Autodesk Fusion 360 part; units mm, degrees
(part 4 of 14)
  arc A924 (85.1535, 49.2252) -> (85.2805, 49.2252) centre (85.217, 49.2252) ccw
  line L1593 (84.034, 50.673) -> (84.584, 50.673)
  arc A925 (84.2645, 50.9778) -> (84.1375, 50.9778) centre (84.201, 50.9778) ccw
  arc A926 (84.2645, 50.9778) -> (84.1375, 50.9778) centre (84.201, 50.9778) ccw
  line L1594 (84.834, 50.9778) -> (84.584, 50.9778)
  line L1595 (84.834, 50.673) -> (85.384, 50.673)
  line L1596 (85.217, 50.9778) -> (85.217, 50.3682)
  arc A927 (84.2645, 49.2252) -> (84.1375, 49.2252) centre (84.201, 49.2252) ccw
  arc A928 (84.1588, 49.23) -> (84.1592, 49.23) centre (84.159, 49.23) ccw
  arc A929 (84.1375, 50.9778) -> (84.2645, 50.9778) centre (84.201, 50.9778) ccw
  arc A930 (85.2805, 50.3682) -> (85.1535, 50.3682) centre (85.217, 50.3682) ccw
  line L1597 (85.259, 49.83) -> (84.159, 49.83)
  arc A931 (85.2805, 49.2252) -> (85.1535, 49.2252) centre (85.217, 49.2252) ccw
  line L1598 (84.034, 50.673) -> (84.584, 50.673)
  line L1599 (84.834, 49.8348) -> (84.584, 49.8348)
  line L1600 (85.259, 49.23) -> (85.259, 49.83)
  line L1601 (84.159, 49.83) -> (84.159, 49.23)
  line L1602 (84.584, 49.2252) -> (84.834, 49.2252)
  line L1603 (84.834, 50.673) -> (85.384, 50.673)
  arc A932 (85.2588, 49.83) -> (85.2592, 49.83) centre (85.259, 49.83) ccw
  line L1604 (84.201, 49.2252) -> (84.201, 49.8348)
  line L1605 (84.034, 49.53) -> (84.584, 49.53)
  arc A933 (84.2645, 50.3682) -> (84.1375, 50.3682) centre (84.201, 50.3682) ccw
  line L1606 (84.584, 50.9778) -> (84.584, 50.3682)
  line L1607 (84.201, 50.9778) -> (85.217, 50.9778)
  arc A934 (84.2645, 50.3682) -> (84.1375, 50.3682) centre (84.201, 50.3682) ccw
  arc A935 (84.1375, 50.3682) -> (84.2645, 50.3682) centre (84.201, 50.3682) ccw
  line L1608 (84.834, 50.3682) -> (84.834, 50.9778)
  arc A936 (84.1375, 49.8348) -> (84.2645, 49.8348) centre (84.201, 49.8348) ccw
  line L1609 (84.034, 49.53) -> (84.584, 49.53)
  arc A937 (85.2805, 50.3682) -> (85.1535, 50.3682) centre (85.217, 50.3682) ccw
  line L1610 (85.217, 49.2252) -> (84.201, 49.2252)
  line L1611 (85.217, 50.3682) -> (84.201, 50.3682)
  line L1612 (84.201, 49.8348) -> (85.217, 49.8348)
  arc A938 (84.1375, 49.2252) -> (84.2645, 49.2252) centre (84.201, 49.2252) ccw
  line L1613 (85.217, 49.8348) -> (85.217, 49.2252)
  arc A939 (84.1588, 49.83) -> (84.1592, 49.83) centre (84.159, 49.83) ccw
  line L1614 (84.834, 50.673) -> (85.384, 50.673)
  line L1615 (84.201, 50.3682) -> (84.201, 50.9778)
  arc A940 (84.1375, 50.9778) -> (84.2645, 50.9778) centre (84.201, 50.9778) ccw
  line L1616 (84.584, 50.3682) -> (84.834, 50.3682)
  arc A941 (85.2805, 49.2252) -> (85.1535, 49.2252) centre (85.217, 49.2252) ccw
  arc A942 (85.1535, 50.3682) -> (85.2805, 50.3682) centre (85.217, 50.3682) ccw
  line L1617 (84.201, 49.8348) -> (85.217, 49.8348)
  arc A943 (84.1592, 49.83) -> (84.1588, 49.83) centre (84.159, 49.83) ccw
  arc A944 (85.2805, 49.8348) -> (85.1535, 49.8348) centre (85.217, 49.8348) ccw
  line L1618 (85.217, 49.8348) -> (85.217, 49.2252)
  line L1619 (84.834, 49.53) -> (85.384, 49.53)
  arc A945 (85.1535, 50.9778) -> (85.2805, 50.9778) centre (85.217, 50.9778) ccw
  arc A946 (85.1535, 49.8348) -> (85.2805, 49.8348) centre (85.217, 49.8348) ccw
  arc A947 (80.818, 55.5408) -> (80.818, 55.5412) centre (80.818, 55.541) ccw
  line L1620 (84.834, 49.53) -> (85.384, 49.53)
  line L1621 (80.518, 54.316) -> (80.518, 54.866)
  line L1622 (80.218, 54.441) -> (80.818, 54.441)
  arc A948 (85.2592, 49.83) -> (85.2588, 49.83) centre (85.259, 49.83) ccw
  arc A949 (80.2132, 54.5465) -> (80.2132, 54.4195) centre (80.2132, 54.483) ccw
  arc A950 (80.8228, 55.4355) -> (80.8228, 55.5625) centre (80.8228, 55.499) ccw
  line L1623 (80.8228, 55.499) -> (80.8228, 54.483)
  line L1624 (80.518, 55.116) -> (80.518, 55.666)
  line L1625 (79.6798, 55.499) -> (79.6798, 54.483)
  arc A951 (80.8228, 55.5625) -> (80.8228, 55.4355) centre (80.8228, 55.499) ccw
  arc A952 (80.218, 55.5408) -> (80.218, 55.5412) centre (80.218, 55.541) ccw
  arc A953 (80.8228, 54.4195) -> (80.8228, 54.5465) centre (80.8228, 54.483) ccw
  arc A954 (80.218, 54.4408) -> (80.218, 54.4412) centre (80.218, 54.441) ccw
  line L1626 (80.8228, 54.866) -> (80.8228, 55.116)
  line L1627 (80.8228, 54.483) -> (80.2132, 54.483)
  arc A955 (80.2132, 54.4195) -> (80.2132, 54.5465) centre (80.2132, 54.483) ccw
  line L1628 (84.834, 49.53) -> (85.384, 49.53)
  arc A956 (80.818, 55.5412) -> (80.818, 55.5408) centre (80.818, 55.541) ccw
  line L1629 (80.218, 55.541) -> (80.218, 54.441)
  line L1630 (79.0702, 55.499) -> (79.6798, 55.499)
  arc A957 (79.6798, 54.5465) -> (79.6798, 54.4195) centre (79.6798, 54.483) ccw
  arc A958 (80.2132, 55.5625) -> (80.2132, 55.4355) centre (80.2132, 55.499) ccw
  line L1631 (79.675, 54.441) -> (79.675, 55.541)
  arc A959 (79.675, 54.4408) -> (79.675, 54.4412) centre (79.675, 54.441) ccw
  line L1632 (79.6798, 54.483) -> (79.0702, 54.483)
  arc A960 (85.1535, 49.2252) -> (85.2805, 49.2252) centre (85.217, 49.2252) ccw
  arc A961 (80.2132, 55.4355) -> (80.2132, 55.5625) centre (80.2132, 55.499) ccw
  line L1633 (80.2132, 54.483) -> (80.2132, 55.499)
  arc A962 (80.8228, 54.4195) -> (80.8228, 54.5465) centre (80.8228, 54.483) ccw
  arc A963 (80.8228, 55.5625) -> (80.8228, 55.4355) centre (80.8228, 55.499) ccw
  arc A964 (80.2132, 54.4195) -> (80.2132, 54.5465) centre (80.2132, 54.483) ccw
  line L1634 (84.834, 49.2252) -> (84.834, 49.8348)
  line L1635 (80.8228, 55.499) -> (80.8228, 54.483)
  line L1636 (80.8228, 55.116) -> (80.2132, 55.116)
  arc A965 (85.1535, 49.8348) -> (85.2805, 49.8348) centre (85.217, 49.8348) ccw
  arc A966 (80.218, 55.5412) -> (80.218, 55.5408) centre (80.218, 55.541) ccw
  arc A967 (80.8228, 54.5465) -> (80.8228, 54.4195) centre (80.8228, 54.483) ccw
  arc A968 (80.2132, 54.5465) -> (80.2132, 54.4195) centre (80.2132, 54.483) ccw
  line L1637 (80.2132, 55.499) -> (80.8228, 55.499)
  arc A969 (84.2645, 49.2252) -> (84.1375, 49.2252) centre (84.201, 49.2252) ccw
  arc A970 (84.2645, 49.8348) -> (84.1375, 49.8348) centre (84.201, 49.8348) ccw
  line L1638 (80.818, 55.541) -> (80.218, 55.541)
  arc A971 (80.818, 54.4408) -> (80.818, 54.4412) centre (80.818, 54.441) ccw
  arc A972 (80.2132, 55.5625) -> (80.2132, 55.4355) centre (80.2132, 55.499) ccw
  line L1639 (80.518, 54.316) -> (80.518, 54.866)
  line L1640 (80.2132, 55.499) -> (80.8228, 55.499)
  line L1641 (80.518, 54.316) -> (80.518, 54.866)
  arc A973 (80.218, 54.4412) -> (80.218, 54.4408) centre (80.218, 54.441) ccw
  line L1642 (80.2132, 54.483) -> (80.2132, 55.499)
  arc A974 (84.2645, 49.8348) -> (84.1375, 49.8348) centre (84.201, 49.8348) ccw
  arc A975 (80.818, 54.4412) -> (80.818, 54.4408) centre (80.818, 54.441) ccw
  line L1643 (80.2132, 54.866) -> (80.8228, 54.866)
  arc A976 (79.0702, 55.4355) -> (79.0702, 55.5625) centre (79.0702, 55.499) ccw
  line L1644 (80.2132, 55.116) -> (80.2132, 54.866)
  arc A977 (80.2132, 55.4355) -> (80.2132, 55.5625) centre (80.2132, 55.499) ccw
  line L1645 (84.159, 49.23) -> (85.259, 49.23)
  arc A978 (84.1592, 49.23) -> (84.1588, 49.23) centre (84.159, 49.23) ccw
  line L1646 (80.8228, 54.483) -> (80.2132, 54.483)
  line L1647 (85.217, 49.2252) -> (84.201, 49.2252)
  arc A979 (85.2805, 49.8348) -> (85.1535, 49.8348) centre (85.217, 49.8348) ccw
  arc A980 (80.8228, 55.4355) -> (80.8228, 55.5625) centre (80.8228, 55.499) ccw
  line L1648 (80.818, 54.441) -> (80.818, 55.541)
  arc A981 (80.8228, 54.5465) -> (80.8228, 54.4195) centre (80.8228, 54.483) ccw
  line L1649 (79.375, 55.116) -> (79.375, 55.666)
  arc A982 (76.1365, 50.3682) -> (76.2635, 50.3682) centre (76.2, 50.3682) ccw
  line L1650 (80.518, 55.116) -> (80.518, 55.666)
  line L1651 (77.258, 50.973) -> (76.158, 50.973)
  arc A983 (79.6798, 55.5625) -> (79.6798, 55.4355) centre (79.6798, 55.499) ccw
  arc A984 (79.075, 54.4412) -> (79.075, 54.4408) centre (79.075, 54.441) ccw
  line L1652 (76.583, 50.3682) -> (76.833, 50.3682)
  arc A985 (77.1525, 50.9778) -> (77.2795, 50.9778) centre (77.216, 50.9778) ccw
  arc A986 (76.1365, 50.9778) -> (76.2635, 50.9778) centre (76.2, 50.9778) ccw
  arc A987 (76.2635, 50.3682) -> (76.1365, 50.3682) centre (76.2, 50.3682) ccw
  arc A988 (79.075, 55.5408) -> (79.075, 55.5412) centre (79.075, 55.541) ccw
  arc A989 (76.2635, 50.3682) -> (76.1365, 50.3682) centre (76.2, 50.3682) ccw
  arc A990 (79.675, 54.4412) -> (79.675, 54.4408) centre (79.675, 54.441) ccw
  line L1653 (76.833, 50.3682) -> (76.833, 50.9778)
  arc A991 (79.0702, 54.4195) -> (79.0702, 54.5465) centre (79.0702, 54.483) ccw
  arc A992 (79.0702, 54.5465) -> (79.0702, 54.4195) centre (79.0702, 54.483) ccw
  line L1654 (76.833, 50.9778) -> (76.583, 50.9778)
  arc A993 (77.2795, 50.3682) -> (77.1525, 50.3682) centre (77.216, 50.3682) ccw
  line L1655 (77.216, 50.3682) -> (76.2, 50.3682)
  arc A994 (77.2578, 50.973) -> (77.2582, 50.973) centre (77.258, 50.973) ccw
  arc A995 (77.2582, 50.373) -> (77.2578, 50.373) centre (77.258, 50.373) ccw
  arc A996 (76.2635, 50.9778) -> (76.1365, 50.9778) centre (76.2, 50.9778) ccw
  arc A997 (76.1582, 50.373) -> (76.1578, 50.373) centre (76.158, 50.373) ccw
  line L1656 (76.583, 50.9778) -> (76.583, 50.3682)
  line L1657 (76.2, 50.9778) -> (77.216, 50.9778)
  arc A998 (76.1365, 50.3682) -> (76.2635, 50.3682) centre (76.2, 50.3682) ccw
  line L1658 (79.6798, 54.483) -> (79.0702, 54.483)
  arc A999 (79.6798, 55.4355) -> (79.6798, 55.5625) centre (79.6798, 55.499) ccw
  line L1659 (79.0702, 54.483) -> (79.0702, 55.499)
  arc A1000 (79.6798, 54.4195) -> (79.6798, 54.5465) centre (79.6798, 54.483) ccw
  line L1660 (76.2, 50.9778) -> (77.216, 50.9778)
  arc A1001 (79.0702, 55.5625) -> (79.0702, 55.4355) centre (79.0702, 55.499) ccw
  line L1661 (79.0702, 54.866) -> (79.6798, 54.866)
  arc A1002 (77.2582, 50.973) -> (77.2578, 50.973) centre (77.258, 50.973) ccw
  line L1662 (79.0702, 55.116) -> (79.0702, 54.866)
  arc A1003 (79.0702, 54.5465) -> (79.0702, 54.4195) centre (79.0702, 54.483) ccw
  arc A1004 (79.675, 55.5412) -> (79.675, 55.5408) centre (79.675, 55.541) ccw
  arc A1005 (79.0702, 55.5625) -> (79.0702, 55.4355) centre (79.0702, 55.499) ccw
  line L1663 (77.216, 50.9778) -> (77.216, 50.3682)
  arc A1006 (77.1525, 50.3682) -> (77.2795, 50.3682) centre (77.216, 50.3682) ccw
  line L1664 (79.675, 55.541) -> (79.075, 55.541)
  arc A1007 (79.0702, 54.4195) -> (79.0702, 54.5465) centre (79.0702, 54.483) ccw
  arc A1008 (79.6798, 54.4195) -> (79.6798, 54.5465) centre (79.6798, 54.483) ccw
  arc A1009 (79.075, 55.5412) -> (79.075, 55.5408) centre (79.075, 55.541) ccw
  line L1665 (79.375, 54.316) -> (79.375, 54.866)
  line L1666 (79.075, 54.441) -> (79.675, 54.441)
  arc A1010 (77.2578, 50.373) -> (77.2582, 50.373) centre (77.258, 50.373) ccw
  line L1667 (76.158, 50.373) -> (77.258, 50.373)
  line L1668 (79.375, 55.116) -> (79.375, 55.666)
  arc A1011 (77.2795, 50.9778) -> (77.1525, 50.9778) centre (77.216, 50.9778) ccw
  line L1669 (79.6798, 55.499) -> (79.6798, 54.483)
  line L1670 (79.6798, 54.866) -> (79.6798, 55.116)
  arc A1012 (79.6798, 55.5625) -> (79.6798, 55.4355) centre (79.6798, 55.499) ccw
  arc A1013 (79.0702, 55.4355) -> (79.0702, 55.5625) centre (79.0702, 55.499) ccw
  arc A1014 (79.075, 54.4408) -> (79.075, 54.4412) centre (79.075, 54.441) ccw
  line L1671 (79.6798, 55.116) -> (79.0702, 55.116)
  arc A1015 (79.6798, 54.5465) -> (79.6798, 54.4195) centre (79.6798, 54.483) ccw
  line L1672 (79.075, 55.541) -> (79.075, 54.441)
  line L1673 (79.0702, 54.483) -> (79.0702, 55.499)
  line L1674 (79.0702, 55.499) -> (79.6798, 55.499)
  line L1675 (80.518, 55.116) -> (80.518, 55.666)
  arc A1016 (79.675, 55.5408) -> (79.675, 55.5412) centre (79.675, 55.541) ccw
  arc A1017 (76.2635, 50.9778) -> (76.1365, 50.9778) centre (76.2, 50.9778) ccw
  arc A1018 (79.6798, 55.4355) -> (79.6798, 55.5625) centre (79.6798, 55.499) ccw
  line L1676 (26.999, 28.694) -> (26.399, 28.694)
  arc A1019 (76.1578, 50.373) -> (76.1582, 50.373) centre (76.158, 50.373) ccw
  arc A1020 (26.399, 28.6943) -> (26.399, 28.6938) centre (26.399, 28.694) ccw
  line L1677 (77.216, 50.3682) -> (76.2, 50.3682)
  line L1678 (79.375, 54.316) -> (79.375, 54.866)
  line L1679 (77.216, 50.9778) -> (77.216, 50.3682)
  line L1680 (26.3942, 27.636) -> (26.3942, 28.652)
  arc A1021 (26.999, 27.5938) -> (26.999, 27.5943) centre (26.999, 27.594) ccw
  arc A1022 (26.399, 27.5938) -> (26.399, 27.5943) centre (26.399, 27.594) ccw
  line L1681 (27.0038, 27.636) -> (26.3942, 27.636)
  arc A1023 (26.999, 28.6938) -> (26.999, 28.6943) centre (26.999, 28.694) ccw
  line L1682 (26.3942, 28.652) -> (27.0038, 28.652)
  line L1683 (76.583, 50.673) -> (76.033, 50.673)
  arc A1024 (27.0038, 27.5725) -> (27.0038, 27.6995) centre (27.0038, 27.636) ccw
  arc A1025 (27.0038, 27.6995) -> (27.0038, 27.5725) centre (27.0038, 27.636) ccw
  line L1684 (26.3942, 28.269) -> (26.3942, 28.019)
  arc A1026 (26.399, 28.6938) -> (26.399, 28.6943) centre (26.399, 28.694) ccw
  line L1685 (82.804, 30.4038) -> (83.82, 30.4038)
  line L1686 (76.583, 50.673) -> (76.033, 50.673)
  arc A1027 (26.3942, 28.5885) -> (26.3942, 28.7155) centre (26.3942, 28.652) ccw
  line L1687 (79.375, 55.116) -> (79.375, 55.666)
  line L1688 (26.999, 27.594) -> (26.999, 28.694)
  line L1689 (26.3942, 28.652) -> (27.0038, 28.652)
  line L1690 (26.399, 27.594) -> (26.999, 27.594)
  line L1691 (26.3942, 27.636) -> (26.3942, 28.652)
  line L1692 (26.699, 28.269) -> (26.699, 28.819)
  arc A1028 (26.3942, 27.5725) -> (26.3942, 27.6995) centre (26.3942, 27.636) ccw
  arc A1029 (83.8622, 29.799) -> (83.8618, 29.799) centre (83.862, 29.799) ccw
  arc A1030 (26.3942, 27.5725) -> (26.3942, 27.6995) centre (26.3942, 27.636) ccw
  line L1693 (76.158, 50.973) -> (76.158, 50.373)
  line L1694 (27.0038, 27.636) -> (26.3942, 27.636)
  arc A1031 (76.1578, 50.973) -> (76.1582, 50.973) centre (76.158, 50.973) ccw
  arc A1032 (27.0038, 28.5885) -> (27.0038, 28.7155) centre (27.0038, 28.652) ccw
  line L1695 (77.383, 50.673) -> (76.833, 50.673)
  line L1696 (76.2, 50.3682) -> (76.2, 50.9778)
  arc A1033 (26.3942, 27.6995) -> (26.3942, 27.5725) centre (26.3942, 27.636) ccw
  arc A1034 (83.8618, 29.799) -> (83.8622, 29.799) centre (83.862, 29.799) ccw
  arc A1035 (77.1525, 50.3682) -> (77.2795, 50.3682) centre (77.216, 50.3682) ccw
  arc A1036 (76.1365, 50.9778) -> (76.2635, 50.9778) centre (76.2, 50.9778) ccw
  arc A1037 (77.2795, 50.3682) -> (77.1525, 50.3682) centre (77.216, 50.3682) ccw
  arc A1038 (26.999, 28.6943) -> (26.999, 28.6938) centre (26.999, 28.694) ccw
  arc A1039 (26.3942, 28.5885) -> (26.3942, 28.7155) centre (26.3942, 28.652) ccw
  arc A1040 (26.999, 27.5943) -> (26.999, 27.5938) centre (26.999, 27.594) ccw
  arc A1041 (26.3942, 28.7155) -> (26.3942, 28.5885) centre (26.3942, 28.652) ccw
  line L1697 (76.583, 50.673) -> (76.033, 50.673)
  line L1698 (26.3942, 28.019) -> (27.0038, 28.019)
  line L1699 (79.375, 54.316) -> (79.375, 54.866)
  arc A1042 (77.1525, 50.9778) -> (77.2795, 50.9778) centre (77.216, 50.9778) ccw
  arc A1043 (27.0038, 27.6995) -> (27.0038, 27.5725) centre (27.0038, 27.636) ccw
  line L1700 (77.383, 50.673) -> (76.833, 50.673)
  arc A1044 (27.0038, 28.5885) -> (27.0038, 28.7155) centre (27.0038, 28.652) ccw
  arc A1045 (76.1582, 50.973) -> (76.1578, 50.973) centre (76.158, 50.973) ccw
  arc A1046 (77.2795, 50.9778) -> (77.1525, 50.9778) centre (77.216, 50.9778) ccw
  arc A1047 (26.399, 27.5943) -> (26.399, 27.5938) centre (26.399, 27.594) ccw
  arc A1048 (27.0038, 27.5725) -> (27.0038, 27.6995) centre (27.0038, 27.636) ccw
  line L1701 (27.0038, 28.652) -> (27.0038, 27.636)
  line L1702 (76.2, 50.3682) -> (76.2, 50.9778)
  line L1703 (26.399, 28.694) -> (26.399, 27.594)
  line L1704 (27.0038, 28.652) -> (27.0038, 27.636)
  line L1705 (77.383, 50.673) -> (76.833, 50.673)
  arc A1049 (26.3942, 28.7155) -> (26.3942, 28.5885) centre (26.3942, 28.652) ccw
  line L1706 (77.258, 50.373) -> (77.258, 50.973)
  arc A1050 (27.0038, 28.7155) -> (27.0038, 28.5885) centre (27.0038, 28.652) ccw
  arc A1051 (27.0038, 28.7155) -> (27.0038, 28.5885) centre (27.0038, 28.652) ccw
  line L1707 (28.1468, 28.652) -> (28.1468, 27.636)
  line L1708 (28.142, 27.594) -> (28.142, 28.694)
  line L1709 (27.542, 28.694) -> (27.542, 27.594)
  line L1710 (82.637, 30.099) -> (83.187, 30.099)
  arc A1052 (82.8675, 29.7942) -> (82.7405, 29.7942) centre (82.804, 29.7942) ccw
  line L1711 (83.187, 30.4038) -> (83.187, 29.7942)
  arc A1053 (82.8675, 30.4038) -> (82.7405, 30.4038) centre (82.804, 30.4038) ccw
  line L1712 (83.82, 29.7942) -> (82.804, 29.7942)
  line L1713 (27.542, 27.594) -> (28.142, 27.594)
  line L1714 (83.82, 29.7942) -> (82.804, 29.7942)
  arc A1054 (83.8618, 30.399) -> (83.8622, 30.399) centre (83.862, 30.399) ccw
  arc A1055 (82.7622, 29.799) -> (82.7618, 29.799) centre (82.762, 29.799) ccw
  line L1715 (83.437, 30.099) -> (83.987, 30.099)
  line L1716 (83.437, 30.099) -> (83.987, 30.099)
  line L1717 (83.437, 30.4038) -> (83.187, 30.4038)
  arc A1056 (83.7565, 29.7942) -> (83.8835, 29.7942) centre (83.82, 29.7942) ccw
  arc A1057 (26.3942, 27.6995) -> (26.3942, 27.5725) centre (26.3942, 27.636) ccw
  arc A1058 (83.7565, 29.7942) -> (83.8835, 29.7942) centre (83.82, 29.7942) ccw
  arc A1059 (82.8675, 29.7942) -> (82.7405, 29.7942) centre (82.804, 29.7942) ccw
  line L1718 (83.82, 30.4038) -> (83.82, 29.7942)
  line L1719 (26.699, 27.469) -> (26.699, 28.019)
  arc A1060 (83.7565, 30.4038) -> (83.8835, 30.4038) centre (83.82, 30.4038) ccw
  line L1720 (26.699, 28.269) -> (26.699, 28.819)
  line L1721 (27.0038, 28.269) -> (26.3942, 28.269)
  line L1722 (83.82, 30.4038) -> (83.82, 29.7942)
  arc A1061 (82.7405, 29.7942) -> (82.8675, 29.7942) centre (82.804, 29.7942) ccw
  arc A1062 (83.7565, 30.4038) -> (83.8835, 30.4038) centre (83.82, 30.4038) ccw
  line L1723 (27.5372, 28.652) -> (28.1468, 28.652)
  line L1724 (28.1468, 27.636) -> (27.5372, 27.636)
  arc A1063 (27.542, 27.5938) -> (27.542, 27.5943) centre (27.542, 27.594) ccw
  line L1725 (28.1468, 27.636) -> (27.5372, 27.636)
  line L1726 (83.862, 29.799) -> (83.862, 30.399)
  arc A1064 (28.1468, 28.5885) -> (28.1468, 28.7155) centre (28.1468, 28.652) ccw
  line L1727 (83.437, 30.099) -> (83.987, 30.099)
  arc A1065 (28.142, 27.5943) -> (28.142, 27.5938) centre (28.142, 27.594) ccw
  arc A1066 (82.7622, 30.399) -> (82.7618, 30.399) centre (82.762, 30.399) ccw
  arc A1067 (27.542, 28.6943) -> (27.542, 28.6938) centre (27.542, 28.694) ccw
  arc A1068 (28.1468, 27.5725) -> (28.1468, 27.6995) centre (28.1468, 27.636) ccw
  line L1728 (82.804, 30.4038) -> (83.82, 30.4038)
  line L1729 (83.862, 30.399) -> (82.762, 30.399)
  arc A1069 (28.142, 27.5938) -> (28.142, 27.5943) centre (28.142, 27.594) ccw
  line L1730 (82.762, 29.799) -> (83.862, 29.799)
  arc A1070 (28.142, 28.6943) -> (28.142, 28.6938) centre (28.142, 28.694) ccw
  line L1731 (82.804, 29.7942) -> (82.804, 30.4038)
  arc A1071 (83.8835, 30.4038) -> (83.7565, 30.4038) centre (83.82, 30.4038) ccw
  arc A1072 (83.8835, 30.4038) -> (83.7565, 30.4038) centre (83.82, 30.4038) ccw
  line L1732 (26.699, 27.469) -> (26.699, 28.019)
  arc A1073 (83.8835, 29.7942) -> (83.7565, 29.7942) centre (83.82, 29.7942) ccw
  arc A1074 (27.542, 28.6938) -> (27.542, 28.6943) centre (27.542, 28.694) ccw
  arc A1075 (28.142, 28.6938) -> (28.142, 28.6943) centre (28.142, 28.694) ccw
  line L1733 (82.637, 30.099) -> (83.187, 30.099)
  line L1734 (27.5372, 27.636) -> (27.5372, 28.652)
  arc A1076 (82.7405, 29.7942) -> (82.8675, 29.7942) centre (82.804, 29.7942) ccw
  line L1735 (26.699, 28.269) -> (26.699, 28.819)
  arc A1077 (82.7618, 29.799) -> (82.7622, 29.799) centre (82.762, 29.799) ccw
  line L1736 (28.142, 28.694) -> (27.542, 28.694)
  arc A1078 (83.8835, 29.7942) -> (83.7565, 29.7942) centre (83.82, 29.7942) ccw
  line L1737 (27.0038, 28.019) -> (27.0038, 28.269)
  line L1738 (82.762, 30.399) -> (82.762, 29.799)
  line L1739 (26.699, 27.469) -> (26.699, 28.019)
  arc A1079 (82.7405, 30.4038) -> (82.8675, 30.4038) centre (82.804, 30.4038) ccw
  arc A1080 (82.7618, 30.399) -> (82.7622, 30.399) centre (82.762, 30.399) ccw
  arc A1081 (83.8622, 30.399) -> (83.8618, 30.399) centre (83.862, 30.399) ccw
  line L1740 (82.804, 29.7942) -> (82.804, 30.4038)
  line L1741 (29.158, 27.594) -> (29.158, 28.694)
  arc A1082 (27.5372, 27.5725) -> (27.5372, 27.6995) centre (27.5372, 27.636) ccw
  arc A1083 (82.7405, 30.4038) -> (82.8675, 30.4038) centre (82.804, 30.4038) ccw
  line L1742 (27.842, 28.269) -> (27.842, 28.819)
  arc A1084 (28.558, 27.5943) -> (28.558, 27.5938) centre (28.558, 27.594) ccw
  line L1743 (27.842, 28.269) -> (27.842, 28.819)
  arc A1085 (28.5532, 28.7155) -> (28.5532, 28.5885) centre (28.5532, 28.652) ccw
  arc A1086 (28.1468, 28.5885) -> (28.1468, 28.7155) centre (28.1468, 28.652) ccw
  line L1744 (83.187, 29.7942) -> (83.437, 29.7942)
  arc A1087 (29.158, 27.5943) -> (29.158, 27.5938) centre (29.158, 27.594) ccw
  line L1745 (27.842, 27.469) -> (27.842, 28.019)
  arc A1088 (82.8675, 30.4038) -> (82.7405, 30.4038) centre (82.804, 30.4038) ccw
  line L1746 (28.558, 28.694) -> (28.558, 27.594)
  line L1747 (29.1628, 27.636) -> (28.5532, 27.636)
  arc A1089 (28.1468, 28.7155) -> (28.1468, 28.5885) centre (28.1468, 28.652) ccw
  arc A1090 (29.158, 28.6943) -> (29.158, 28.6938) centre (29.158, 28.694) ccw
  arc A1091 (28.558, 27.5938) -> (28.558, 27.5943) centre (28.558, 27.594) ccw
  arc A1092 (27.5372, 28.7155) -> (27.5372, 28.5885) centre (27.5372, 28.652) ccw
  line L1748 (28.1468, 28.019) -> (28.1468, 28.269)
  arc A1093 (28.5532, 27.5725) -> (28.5532, 27.6995) centre (28.5532, 27.636) ccw
  line L1749 (28.558, 27.594) -> (29.158, 27.594)
  arc A1094 (27.542, 27.5943) -> (27.542, 27.5938) centre (27.542, 27.594) ccw
  line L1750 (28.5532, 28.652) -> (29.1628, 28.652)
  line L1751 (82.637, 30.099) -> (83.187, 30.099)
  line L1752 (29.701, 28.694) -> (29.701, 27.594)
  arc A1095 (30.301, 27.5943) -> (30.301, 27.5938) centre (30.301, 27.594) ccw
  arc A1096 (28.5532, 27.6995) -> (28.5532, 27.5725) centre (28.5532, 27.636) ccw
  arc A1097 (28.5532, 27.5725) -> (28.5532, 27.6995) centre (28.5532, 27.636) ccw
  arc A1098 (29.1628, 27.6995) -> (29.1628, 27.5725) centre (29.1628, 27.636) ccw
  line L1753 (29.1628, 28.019) -> (29.1628, 28.269)
  line L1754 (28.5532, 28.269) -> (28.5532, 28.019)
  line L1755 (29.701, 27.594) -> (30.301, 27.594)
  line L1756 (28.858, 28.269) -> (28.858, 28.819)
  line L1757 (28.1468, 28.652) -> (28.1468, 27.636)
  line L1758 (29.158, 28.694) -> (28.558, 28.694)
  arc A1099 (29.1628, 28.7155) -> (29.1628, 28.5885) centre (29.1628, 28.652) ccw
  arc A1100 (28.1468, 28.7155) -> (28.1468, 28.5885) centre (28.1468, 28.652) ccw
  line L1759 (27.5372, 28.652) -> (28.1468, 28.652)
  arc A1101 (28.558, 28.6943) -> (28.558, 28.6938) centre (28.558, 28.694) ccw
  arc A1102 (27.5372, 27.6995) -> (27.5372, 27.5725) centre (27.5372, 27.636) ccw
  line L1760 (83.437, 29.7942) -> (83.437, 30.4038)
  arc A1103 (27.5372, 28.5885) -> (27.5372, 28.7155) centre (27.5372, 28.652) ccw
  line L1761 (27.5372, 28.269) -> (27.5372, 28.019)
  line L1762 (27.5372, 28.019) -> (28.1468, 28.019)
  arc A1104 (28.1468, 27.6995) -> (28.1468, 27.5725) centre (28.1468, 27.636) ccw
  arc A1105 (27.5372, 28.7155) -> (27.5372, 28.5885) centre (27.5372, 28.652) ccw
  line L1763 (27.842, 28.269) -> (27.842, 28.819)
  arc A1106 (29.158, 27.5938) -> (29.158, 27.5943) centre (29.158, 27.594) ccw
  arc A1107 (28.558, 28.6938) -> (28.558, 28.6943) centre (28.558, 28.694) ccw
  arc A1108 (29.1628, 27.5725) -> (29.1628, 27.6995) centre (29.1628, 27.636) ccw
  line L1764 (27.5372, 27.636) -> (27.5372, 28.652)
  arc A1109 (27.5372, 28.5885) -> (27.5372, 28.7155) centre (27.5372, 28.652) ccw
  arc A1110 (29.1628, 28.5885) -> (29.1628, 28.7155) centre (29.1628, 28.652) ccw
  line L1765 (27.842, 27.469) -> (27.842, 28.019)
  arc A1111 (27.5372, 27.5725) -> (27.5372, 27.6995) centre (27.5372, 27.636) ccw
  arc A1112 (28.1468, 27.6995) -> (28.1468, 27.5725) centre (28.1468, 27.636) ccw
  arc A1113 (28.5532, 28.5885) -> (28.5532, 28.7155) centre (28.5532, 28.652) ccw
  line L1766 (29.1628, 28.652) -> (29.1628, 27.636)
  arc A1114 (28.1468, 27.5725) -> (28.1468, 27.6995) centre (28.1468, 27.636) ccw
  line L1767 (28.5532, 27.636) -> (28.5532, 28.652)
  arc A1115 (29.158, 28.6938) -> (29.158, 28.6943) centre (29.158, 28.694) ccw
  line L1768 (27.842, 27.469) -> (27.842, 28.019)
  arc A1116 (27.5372, 27.6995) -> (27.5372, 27.5725) centre (27.5372, 27.636) ccw
  line L1769 (28.1468, 28.269) -> (27.5372, 28.269)
  line L1770 (30.001, 28.269) -> (30.001, 28.819)
  line L1771 (30.3058, 28.652) -> (30.3058, 27.636)
  arc A1117 (29.6962, 28.7155) -> (29.6962, 28.5885) centre (29.6962, 28.652) ccw
  line L1772 (28.858, 27.469) -> (28.858, 28.019)
  arc A1118 (29.1628, 28.5885) -> (29.1628, 28.7155) centre (29.1628, 28.652) ccw
  line L1773 (29.1628, 28.652) -> (29.1628, 27.636)
  arc A1119 (31.444, 27.5938) -> (31.444, 27.5943) centre (31.444, 27.594) ccw
  line L1774 (30.001, 28.269) -> (30.001, 28.819)
  line L1775 (29.6962, 28.269) -> (29.6962, 28.019)
  line L1776 (31.444, 28.694) -> (30.844, 28.694)
  arc A1120 (30.301, 27.5938) -> (30.301, 27.5943) centre (30.301, 27.594) ccw
  line L1777 (30.3058, 28.269) -> (29.6962, 28.269)
  line L1778 (30.001, 27.469) -> (30.001, 28.019)
  arc A1121 (31.444, 27.5943) -> (31.444, 27.5938) centre (31.444, 27.594) ccw
  line L1779 (30.3058, 28.019) -> (30.3058, 28.269)
  arc A1122 (30.844, 27.5943) -> (30.844, 27.5938) centre (30.844, 27.594) ccw
  arc A1123 (31.444, 28.6938) -> (31.444, 28.6943) centre (31.444, 28.694) ccw
  line L1780 (30.844, 28.694) -> (30.844, 27.594)
  line L1781 (30.3058, 27.636) -> (29.6962, 27.636)
  line L1782 (30.001, 27.469) -> (30.001, 28.019)
  arc A1124 (29.1628, 27.5725) -> (29.1628, 27.6995) centre (29.1628, 27.636) ccw
  arc A1125 (30.301, 28.6938) -> (30.301, 28.6943) centre (30.301, 28.694) ccw
  arc A1126 (29.701, 27.5943) -> (29.701, 27.5938) centre (29.701, 27.594) ccw
  arc A1127 (29.6962, 27.5725) -> (29.6962, 27.6995) centre (29.6962, 27.636) ccw
  arc A1128 (30.3058, 28.5885) -> (30.3058, 28.7155) centre (30.3058, 28.652) ccw
  arc A1129 (30.844, 28.6938) -> (30.844, 28.6943) centre (30.844, 28.694) ccw
  line L1783 (28.5532, 28.652) -> (29.1628, 28.652)
  line L1784 (29.6962, 28.652) -> (30.3058, 28.652)
  arc A1130 (30.844, 28.6943) -> (30.844, 28.6938) centre (30.844, 28.694) ccw
  arc A1131 (28.5532, 28.5885) -> (28.5532, 28.7155) centre (28.5532, 28.652) ccw
  line L1785 (29.1628, 27.636) -> (28.5532, 27.636)
  line L1786 (28.5532, 28.019) -> (29.1628, 28.019)
  line L1787 (31.444, 27.594) -> (31.444, 28.694)
  arc A1132 (30.3058, 27.6995) -> (30.3058, 27.5725) centre (30.3058, 27.636) ccw
  line L1788 (28.858, 27.469) -> (28.858, 28.019)
  arc A1133 (29.701, 27.5938) -> (29.701, 27.5943) centre (29.701, 27.594) ccw
  arc A1134 (29.6962, 27.5725) -> (29.6962, 27.6995) centre (29.6962, 27.636) ccw
  line L1789 (28.858, 28.269) -> (28.858, 28.819)
  line L1790 (29.6962, 27.636) -> (29.6962, 28.652)
  line L1791 (30.301, 27.594) -> (30.301, 28.694)
  line L1792 (28.858, 27.469) -> (28.858, 28.019)
  line L1793 (29.1628, 28.269) -> (28.5532, 28.269)
  arc A1135 (29.6962, 28.5885) -> (29.6962, 28.7155) centre (29.6962, 28.652) ccw
  arc A1136 (29.701, 28.6943) -> (29.701, 28.6938) centre (29.701, 28.694) ccw
  arc A1137 (30.3058, 27.5725) -> (30.3058, 27.6995) centre (30.3058, 27.636) ccw
  line L1794 (28.858, 28.269) -> (28.858, 28.819)
  arc A1138 (30.3058, 28.5885) -> (30.3058, 28.7155) centre (30.3058, 28.652) ccw
  line L1795 (30.3058, 27.636) -> (29.6962, 27.636)
  line L1796 (28.5532, 27.636) -> (28.5532, 28.652)
  arc A1139 (28.5532, 28.7155) -> (28.5532, 28.5885) centre (28.5532, 28.652) ccw
  arc A1140 (29.1628, 27.6995) -> (29.1628, 27.5725) centre (29.1628, 27.636) ccw
  arc A1141 (30.301, 28.6943) -> (30.301, 28.6938) centre (30.301, 28.694) ccw
  arc A1142 (28.5532, 27.6995) -> (28.5532, 27.5725) centre (28.5532, 27.636) ccw
  line L1797 (30.301, 28.694) -> (29.701, 28.694)
  line L1798 (30.3058, 28.652) -> (30.3058, 27.636)
  arc A1143 (29.6962, 28.5885) -> (29.6962, 28.7155) centre (29.6962, 28.652) ccw
  arc A1144 (29.1628, 28.7155) -> (29.1628, 28.5885) centre (29.1628, 28.652) ccw
  arc A1145 (29.701, 28.6938) -> (29.701, 28.6943) centre (29.701, 28.694) ccw
  line L1799 (29.6962, 27.636) -> (29.6962, 28.652)
  arc A1146 (29.6962, 27.6995) -> (29.6962, 27.5725) centre (29.6962, 27.636) ccw
  line L1800 (29.6962, 28.652) -> (30.3058, 28.652)
  arc A1147 (30.3058, 28.7155) -> (30.3058, 28.5885) centre (30.3058, 28.652) ccw
  arc A1148 (31.4488, 27.5725) -> (31.4488, 27.6995) centre (31.4488, 27.636) ccw
  arc A1149 (30.3058, 27.5725) -> (30.3058, 27.6995) centre (30.3058, 27.636) ccw
  arc A1150 (30.8392, 28.5885) -> (30.8392, 28.7155) centre (30.8392, 28.652) ccw
  line L1801 (31.4488, 27.636) -> (30.8392, 27.636)
  line L1802 (31.4488, 28.652) -> (31.4488, 27.636)
  arc A1151 (30.3058, 28.7155) -> (30.3058, 28.5885) centre (30.3058, 28.652) ccw
  line L1803 (31.144, 28.269) -> (31.144, 28.819)
  arc A1152 (32.587, 27.5943) -> (32.587, 27.5938) centre (32.587, 27.594) ccw
  line L1804 (32.587, 27.594) -> (32.587, 28.694)
  arc A1153 (31.4488, 27.5725) -> (31.4488, 27.6995) centre (31.4488, 27.636) ccw
  arc A1154 (31.4488, 27.6995) -> (31.4488, 27.5725) centre (31.4488, 27.636) ccw
  arc A1155 (30.8392, 27.6995) -> (30.8392, 27.5725) centre (30.8392, 27.636) ccw
  arc A1156 (31.987, 28.6943) -> (31.987, 28.6938) centre (31.987, 28.694) ccw
  line L1805 (32.5918, 28.652) -> (32.5918, 27.636)
  line L1806 (30.8392, 28.019) -> (31.4488, 28.019)
  line L1807 (32.5918, 28.652) -> (32.5918, 27.636)
  arc A1157 (31.4488, 27.6995) -> (31.4488, 27.5725) centre (31.4488, 27.636) ccw
  line L1808 (32.5918, 27.636) -> (31.9822, 27.636)
  line L1809 (31.987, 28.694) -> (31.987, 27.594)
  line L1810 (31.144, 28.269) -> (31.144, 28.819)
  arc A1158 (30.8392, 27.5725) -> (30.8392, 27.6995) centre (30.8392, 27.636) ccw
  line L1811 (31.144, 27.469) -> (31.144, 28.019)
  line L1812 (32.587, 28.694) -> (31.987, 28.694)
  arc A1159 (30.8392, 28.7155) -> (30.8392, 28.5885) centre (30.8392, 28.652) ccw
  line L1813 (31.144, 28.269) -> (31.144, 28.819)
  arc A1160 (29.926, 31.4108) -> (29.926, 31.4112) centre (29.926, 31.411) ccw
  line L1814 (31.4488, 28.019) -> (31.4488, 28.269)
  line L1815 (29.926, 31.411) -> (29.926, 30.311)
  arc A1161 (31.9822, 28.5885) -> (31.9822, 28.7155) centre (31.9822, 28.652) ccw
  arc A1162 (31.4488, 28.5885) -> (31.4488, 28.7155) centre (31.4488, 28.652) ccw
  line L1816 (30.8392, 27.636) -> (30.8392, 28.652)
  line L1817 (31.4488, 28.652) -> (31.4488, 27.636)
  arc A1163 (31.4488, 28.5885) -> (31.4488, 28.7155) centre (31.4488, 28.652) ccw
  arc A1164 (31.987, 27.5938) -> (31.987, 27.5943) centre (31.987, 27.594) ccw
  arc A1165 (29.6962, 27.6995) -> (29.6962, 27.5725) centre (29.6962, 27.636) ccw
  line L1818 (31.4488, 28.269) -> (30.8392, 28.269)
  line L1819 (31.9822, 28.652) -> (32.5918, 28.652)
  arc A1166 (30.3058, 27.6995) -> (30.3058, 27.5725) centre (30.3058, 27.636) ccw
  line L1820 (29.6962, 28.019) -> (30.3058, 28.019)
  line L1821 (30.8392, 27.636) -> (30.8392, 28.652)
  line L1822 (31.987, 27.594) -> (32.587, 27.594)
  line L1823 (31.144, 27.469) -> (31.144, 28.019)
  line L1824 (31.144, 27.469) -> (31.144, 28.019)
  line L1825 (31.4488, 27.636) -> (30.8392, 27.636)
  arc A1167 (32.587, 27.5938) -> (32.587, 27.5943) centre (32.587, 27.594) ccw
  arc A1168 (31.4488, 28.7155) -> (31.4488, 28.5885) centre (31.4488, 28.652) ccw
  arc A1169 (30.844, 27.5938) -> (30.844, 27.5943) centre (30.844, 27.594) ccw
  arc A1170 (31.444, 28.6943) -> (31.444, 28.6938) centre (31.444, 28.694) ccw
  line L1826 (30.8392, 28.652) -> (31.4488, 28.652)
  arc A1171 (31.4488, 28.7155) -> (31.4488, 28.5885) centre (31.4488, 28.652) ccw
  line L1827 (30.8392, 28.652) -> (31.4488, 28.652)
  line L1828 (30.001, 28.269) -> (30.001, 28.819)
  arc A1172 (29.6962, 28.7155) -> (29.6962, 28.5885) centre (29.6962, 28.652) ccw
  line L1829 (30.8392, 28.269) -> (30.8392, 28.019)
  arc A1173 (32.587, 28.6943) -> (32.587, 28.6938) centre (32.587, 28.694) ccw
  arc A1174 (32.587, 28.6938) -> (32.587, 28.6943) centre (32.587, 28.694) ccw
  line L1830 (30.844, 27.594) -> (31.444, 27.594)
  arc A1175 (30.8392, 27.5725) -> (30.8392, 27.6995) centre (30.8392, 27.636) ccw
  arc A1176 (30.8392, 27.6995) -> (30.8392, 27.5725) centre (30.8392, 27.636) ccw
  arc A1177 (30.8392, 28.7155) -> (30.8392, 28.5885) centre (30.8392, 28.652) ccw
  arc A1178 (30.8392, 28.5885) -> (30.8392, 28.7155) centre (30.8392, 28.652) ccw
  line L1831 (30.001, 27.469) -> (30.001, 28.019)
  arc A1179 (31.987, 28.6938) -> (31.987, 28.6943) centre (31.987, 28.694) ccw
  arc A1180 (31.987, 27.5943) -> (31.987, 27.5938) centre (31.987, 27.594) ccw
  line L1832 (29.9212, 30.353) -> (29.9212, 31.369)
  line L1833 (32.287, 27.469) -> (32.287, 28.019)
  arc A1181 (32.5918, 28.5885) -> (32.5918, 28.7155) centre (32.5918, 28.652) ccw
  arc A1182 (32.5918, 28.5885) -> (32.5918, 28.7155) centre (32.5918, 28.652) ccw
  line L1834 (31.9822, 27.636) -> (31.9822, 28.652)
  arc A1183 (31.9822, 28.7155) -> (31.9822, 28.5885) centre (31.9822, 28.652) ccw
  arc A1184 (29.9212, 30.4165) -> (29.9212, 30.2895) centre (29.9212, 30.353) ccw
  arc A1185 (30.526, 31.4112) -> (30.526, 31.4108) centre (30.526, 31.411) ccw
  line L1835 (32.287, 27.469) -> (32.287, 28.019)
  arc A1186 (31.9822, 27.6995) -> (31.9822, 27.5725) centre (31.9822, 27.636) ccw
  line L1836 (30.226, 31.536) -> (30.226, 30.986)
  arc A1187 (31.9822, 28.7155) -> (31.9822, 28.5885) centre (31.9822, 28.652) ccw
  arc A1188 (29.9212, 30.4165) -> (29.9212, 30.2895) centre (29.9212, 30.353) ccw
  line L1837 (30.226, 31.536) -> (30.226, 30.986)
  line L1838 (31.069, 31.411) -> (31.069, 30.311)
  line L1839 (30.226, 31.536) -> (30.226, 30.986)
  arc A1189 (29.9212, 31.4325) -> (29.9212, 31.3055) centre (29.9212, 31.369) ccw
  arc A1190 (29.926, 30.3112) -> (29.926, 30.3108) centre (29.926, 30.311) ccw
  line L1840 (29.9212, 31.369) -> (30.5308, 31.369)
  arc A1191 (30.5308, 31.4325) -> (30.5308, 31.3055) centre (30.5308, 31.369) ccw
  line L1841 (32.287, 27.469) -> (32.287, 28.019)
  line L1842 (32.5918, 28.019) -> (32.5918, 28.269)
  arc A1192 (30.526, 31.4108) -> (30.526, 31.4112) centre (30.526, 31.411) ccw
  line L1843 (31.9822, 28.019) -> (32.5918, 28.019)
  arc A1193 (32.5918, 28.7155) -> (32.5918, 28.5885) centre (32.5918, 28.652) ccw
  arc A1194 (32.5918, 27.6995) -> (32.5918, 27.5725) centre (32.5918, 27.636) ccw
  arc A1195 (29.9212, 31.3055) -> (29.9212, 31.4325) centre (29.9212, 31.369) ccw
  line L1844 (29.9212, 30.736) -> (30.5308, 30.736)
  arc A1196 (29.9212, 30.2895) -> (29.9212, 30.4165) centre (29.9212, 30.353) ccw
  line L1845 (30.226, 30.736) -> (30.226, 30.186)
  arc A1197 (30.5308, 30.4165) -> (30.5308, 30.2895) centre (30.5308, 30.353) ccw
  line L1846 (30.226, 30.736) -> (30.226, 30.186)
  line L1847 (29.9212, 30.353) -> (29.9212, 31.369)
  line L1848 (30.526, 31.411) -> (29.926, 31.411)
  arc A1198 (29.9212, 31.4325) -> (29.9212, 31.3055) centre (29.9212, 31.369) ccw
  line L1849 (31.069, 30.311) -> (31.669, 30.311)
  line L1850 (31.9822, 28.269) -> (31.9822, 28.019)
  line L1851 (32.287, 28.269) -> (32.287, 28.819)
  line L1852 (29.926, 30.311) -> (30.526, 30.311)
  line L1853 (31.9822, 27.636) -> (31.9822, 28.652)
  arc A1199 (32.5918, 27.5725) -> (32.5918, 27.6995) centre (32.5918, 27.636) ccw
  line L1854 (32.5918, 27.636) -> (31.9822, 27.636)
  line L1855 (31.9822, 28.652) -> (32.5918, 28.652)
  line L1856 (29.9212, 30.986) -> (29.9212, 30.736)
  line L1857 (32.287, 28.269) -> (32.287, 28.819)
  line L1858 (30.5308, 30.736) -> (30.5308, 30.986)
  arc A1200 (29.9212, 31.3055) -> (29.9212, 31.4325) centre (29.9212, 31.369) ccw
  arc A1201 (31.9822, 28.5885) -> (31.9822, 28.7155) centre (31.9822, 28.652) ccw
  line L1859 (32.5918, 28.269) -> (31.9822, 28.269)
  line L1860 (30.5308, 30.353) -> (29.9212, 30.353)
  arc A1202 (31.9822, 27.5725) -> (31.9822, 27.6995) centre (31.9822, 27.636) ccw
  line L1861 (30.526, 30.311) -> (30.526, 31.411)
  arc A1203 (31.9822, 27.5725) -> (31.9822, 27.6995) centre (31.9822, 27.636) ccw
  line L1862 (32.287, 28.269) -> (32.287, 28.819)
  arc A1204 (31.9822, 27.6995) -> (31.9822, 27.5725) centre (31.9822, 27.636) ccw
  arc A1205 (29.926, 31.4112) -> (29.926, 31.4108) centre (29.926, 31.411) ccw
  arc A1206 (30.5308, 31.3055) -> (30.5308, 31.4325) centre (30.5308, 31.369) ccw
  arc A1207 (32.5918, 28.7155) -> (32.5918, 28.5885) centre (32.5918, 28.652) ccw
  line L1863 (30.5308, 30.353) -> (29.9212, 30.353)
  line L1864 (30.226, 30.736) -> (30.226, 30.186)
  arc A1208 (32.5918, 27.5725) -> (32.5918, 27.6995) centre (32.5918, 27.636) ccw
  arc A1209 (29.9212, 30.2895) -> (29.9212, 30.4165) centre (29.9212, 30.353) ccw
  arc A1210 (32.5918, 27.6995) -> (32.5918, 27.5725) centre (32.5918, 27.636) ccw
  arc A1211 (30.526, 30.3108) -> (30.526, 30.3112) centre (30.526, 30.311) ccw
  arc A1212 (31.669, 30.3108) -> (31.669, 30.3112) centre (31.669, 30.311) ccw
  line L1865 (31.369, 31.536) -> (31.369, 30.986)
  line L1866 (31.369, 30.736) -> (31.369, 30.186)
  line L1867 (31.6738, 30.353) -> (31.0642, 30.353)
  arc A1213 (31.069, 31.4112) -> (31.069, 31.4108) centre (31.069, 31.411) ccw
  arc A1214 (21.1455, 32.0802) -> (21.2725, 32.0802) centre (21.209, 32.0802) ccw
  line L1868 (29.9212, 31.369) -> (30.5308, 31.369)
  arc A1215 (30.5308, 30.2895) -> (30.5308, 30.4165) centre (30.5308, 30.353) ccw
  line L1869 (31.6738, 31.369) -> (31.6738, 30.353)
  line L1870 (31.369, 31.536) -> (31.369, 30.986)
  arc A1216 (31.069, 30.3108) -> (31.069, 30.3112) centre (31.069, 30.311) ccw
  line L1871 (31.669, 30.311) -> (31.669, 31.411)
  arc A1217 (30.5308, 31.4325) -> (30.5308, 31.3055) centre (30.5308, 31.369) ccw
  line L1872 (31.0642, 30.353) -> (31.0642, 31.369)
  arc A1218 (31.6738, 30.2895) -> (31.6738, 30.4165) centre (31.6738, 30.353) ccw
  line L1873 (31.6738, 31.369) -> (31.6738, 30.353)
  line L1874 (30.5308, 31.369) -> (30.5308, 30.353)
  arc A1219 (30.5308, 30.2895) -> (30.5308, 30.4165) centre (30.5308, 30.353) ccw
  arc A1220 (31.069, 30.3112) -> (31.069, 30.3108) centre (31.069, 30.311) ccw
  line L1875 (31.369, 30.736) -> (31.369, 30.186)
  arc A1221 (31.6738, 31.4325) -> (31.6738, 31.3055) centre (31.6738, 31.369) ccw
  arc A1222 (31.6738, 30.4165) -> (31.6738, 30.2895) centre (31.6738, 30.353) ccw
  arc A1223 (31.0642, 30.4165) -> (31.0642, 30.2895) centre (31.0642, 30.353) ccw
  arc A1224 (31.0642, 30.2895) -> (31.0642, 30.4165) centre (31.0642, 30.353) ccw
  arc A1225 (31.6738, 31.4325) -> (31.6738, 31.3055) centre (31.6738, 31.369) ccw
  line L1876 (21.209, 32.6898) -> (21.209, 32.0802)
  line L1877 (20.193, 32.6898) -> (21.209, 32.6898)
  arc A1226 (20.2565, 32.0802) -> (20.1295, 32.0802) centre (20.193, 32.0802) ccw
  line L1878 (31.369, 30.736) -> (31.369, 30.186)
  arc A1227 (21.2725, 32.0802) -> (21.1455, 32.0802) centre (21.209, 32.0802) ccw
  line L1879 (21.376, 32.385) -> (20.826, 32.385)
  arc A1228 (31.0642, 31.3055) -> (31.0642, 31.4325) centre (31.0642, 31.369) ccw
  arc A1229 (31.0642, 31.4325) -> (31.0642, 31.3055) centre (31.0642, 31.369) ccw
  arc A1230 (20.1508, 32.085) -> (20.1512, 32.085) centre (20.151, 32.085) ccw
  line L1880 (31.6738, 30.986) -> (31.0642, 30.986)
  arc A1231 (21.2512, 32.085) -> (21.2508, 32.085) centre (21.251, 32.085) ccw
  arc A1232 (20.1295, 32.6898) -> (20.2565, 32.6898) centre (20.193, 32.6898) ccw
  line L1881 (30.5308, 30.986) -> (29.9212, 30.986)
  arc A1233 (31.0642, 30.4165) -> (31.0642, 30.2895) centre (31.0642, 30.353) ccw
  arc A1234 (30.526, 30.3112) -> (30.526, 30.3108) centre (30.526, 30.311) ccw
  arc A1235 (31.0642, 31.3055) -> (31.0642, 31.4325) centre (31.0642, 31.369) ccw
  arc A1236 (30.5308, 30.4165) -> (30.5308, 30.2895) centre (30.5308, 30.353) ccw
  line L1882 (31.6738, 30.736) -> (31.6738, 30.986)
  line L1883 (30.5308, 31.369) -> (30.5308, 30.353)
  line L1884 (31.669, 31.411) -> (31.069, 31.411)
  arc A1237 (31.6738, 30.2895) -> (31.6738, 30.4165) centre (31.6738, 30.353) ccw
  line L1885 (31.369, 31.536) -> (31.369, 30.986)
  arc A1238 (31.669, 31.4108) -> (31.669, 31.4112) centre (31.669, 31.411) ccw
  line L1886 (31.0642, 30.736) -> (31.6738, 30.736)
  arc A1239 (31.069, 31.4108) -> (31.069, 31.4112) centre (31.069, 31.411) ccw
  arc A1240 (31.669, 31.4112) -> (31.669, 31.4108) centre (31.669, 31.411) ccw
  arc A1241 (29.926, 30.3108) -> (29.926, 30.3112) centre (29.926, 30.311) ccw
  line L1887 (31.0642, 30.353) -> (31.0642, 31.369)
  line L1888 (31.0642, 31.369) -> (31.6738, 31.369)
  arc A1242 (31.0642, 31.4325) -> (31.0642, 31.3055) centre (31.0642, 31.369) ccw
  arc A1243 (31.6738, 31.3055) -> (31.6738, 31.4325) centre (31.6738, 31.369) ccw
  line L1889 (31.6738, 30.353) -> (31.0642, 30.353)
  line L1890 (31.0642, 30.986) -> (31.0642, 30.736)
  arc A1244 (31.6738, 31.3055) -> (31.6738, 31.4325) centre (31.6738, 31.369) ccw
  line L1891 (31.0642, 31.369) -> (31.6738, 31.369)
  arc A1245 (31.0642, 30.2895) -> (31.0642, 30.4165) centre (31.0642, 30.353) ccw
  arc A1246 (31.669, 30.3112) -> (31.669, 30.3108) centre (31.669, 30.311) ccw
  arc A1247 (30.5308, 31.3055) -> (30.5308, 31.4325) centre (30.5308, 31.369) ccw
  arc A1248 (31.6738, 30.4165) -> (31.6738, 30.2895) centre (31.6738, 30.353) ccw
  arc A1249 (21.2725, 32.0802) -> (21.1455, 32.0802) centre (21.209, 32.0802) ccw
  line L1892 (34.255, 56.7108) -> (34.255, 56.1012)
  arc A1250 (34.1915, 56.1012) -> (34.3185, 56.1012) centre (34.255, 56.1012) ccw
  arc A1251 (34.3185, 56.1012) -> (34.1915, 56.1012) centre (34.255, 56.1012) ccw
  arc A1252 (33.1755, 56.1012) -> (33.3025, 56.1012) centre (33.239, 56.1012) ccw
  line L1893 (20.151, 32.085) -> (21.251, 32.085)
  line L1894 (21.251, 32.685) -> (20.151, 32.685)
  arc A1253 (20.1508, 32.685) -> (20.1512, 32.685) centre (20.151, 32.685) ccw
  arc A1254 (21.2508, 32.685) -> (21.2512, 32.685) centre (21.251, 32.685) ccw
  line L1895 (20.193, 32.6898) -> (21.209, 32.6898)
  arc A1255 (34.2967, 56.706) -> (34.2972, 56.706) centre (34.297, 56.706) ccw
  arc A1256 (33.1967, 56.106) -> (33.1972, 56.106) centre (33.197, 56.106) ccw
  arc A1257 (34.1915, 56.1012) -> (34.3185, 56.1012) centre (34.255, 56.1012) ccw
  arc A1258 (33.1755, 56.1012) -> (33.3025, 56.1012) centre (33.239, 56.1012) ccw
  arc A1259 (34.3185, 56.7108) -> (34.1915, 56.7108) centre (34.255, 56.7108) ccw
  line L1896 (20.576, 32.385) -> (20.026, 32.385)
  line L1897 (21.209, 32.0802) -> (20.193, 32.0802)
  line L1898 (20.576, 32.6898) -> (20.576, 32.0802)
  line L1899 (21.251, 32.085) -> (21.251, 32.685)
  arc A1260 (21.2508, 32.085) -> (21.2512, 32.085) centre (21.251, 32.085) ccw
  arc A1261 (21.1455, 32.6898) -> (21.2725, 32.6898) centre (21.209, 32.6898) ccw
  arc A1262 (20.1295, 32.0802) -> (20.2565, 32.0802) centre (20.193, 32.0802) ccw
  line L1900 (34.422, 56.406) -> (33.872, 56.406)
  line L1901 (34.422, 56.406) -> (33.872, 56.406)
  line L1902 (20.826, 32.6898) -> (20.576, 32.6898)
  line L1903 (33.239, 56.1012) -> (33.239, 56.7108)
  line L1904 (34.297, 56.106) -> (34.297, 56.706)
  arc A1263 (21.2725, 32.6898) -> (21.1455, 32.6898) centre (21.209, 32.6898) ccw
  line L1905 (33.239, 56.7108) -> (34.255, 56.7108)
  arc A1264 (34.3185, 56.1012) -> (34.1915, 56.1012) centre (34.255, 56.1012) ccw
  arc A1265 (20.1512, 32.085) -> (20.1508, 32.085) centre (20.151, 32.085) ccw
  arc A1266 (21.2725, 32.6898) -> (21.1455, 32.6898) centre (21.209, 32.6898) ccw
  arc A1267 (34.2972, 56.706) -> (34.2967, 56.706) centre (34.297, 56.706) ccw
  line L1906 (21.376, 32.385) -> (20.826, 32.385)
  arc A1268 (20.2565, 32.6898) -> (20.1295, 32.6898) centre (20.193, 32.6898) ccw
  line L1907 (20.151, 32.685) -> (20.151, 32.085)
  line L1908 (20.193, 32.0802) -> (20.193, 32.6898)
  arc A1269 (21.1455, 32.6898) -> (21.2725, 32.6898) centre (21.209, 32.6898) ccw
  line L1909 (20.193, 32.0802) -> (20.193, 32.6898)
  arc A1270 (21.1455, 32.0802) -> (21.2725, 32.0802) centre (21.209, 32.0802) ccw
  arc A1271 (20.1295, 32.0802) -> (20.2565, 32.0802) centre (20.193, 32.0802) ccw
  line L1910 (20.576, 32.0802) -> (20.826, 32.0802)
  arc A1272 (20.2565, 32.0802) -> (20.1295, 32.0802) centre (20.193, 32.0802) ccw
  arc A1273 (20.1295, 32.6898) -> (20.2565, 32.6898) centre (20.193, 32.6898) ccw
  line L1911 (21.209, 32.6898) -> (21.209, 32.0802)
  arc A1274 (20.1512, 32.685) -> (20.1508, 32.685) centre (20.151, 32.685) ccw
  line L1912 (33.197, 56.706) -> (33.197, 56.106)
  arc A1275 (20.2565, 32.6898) -> (20.1295, 32.6898) centre (20.193, 32.6898) ccw
  line L1913 (21.209, 32.0802) -> (20.193, 32.0802)
  line L1914 (21.376, 32.385) -> (20.826, 32.385)
  line L1915 (20.826, 32.0802) -> (20.826, 32.6898)
  line L1916 (33.197, 56.106) -> (34.297, 56.106)
  arc A1276 (21.2512, 32.685) -> (21.2508, 32.685) centre (21.251, 32.685) ccw
  line L1917 (77.216, 51.6382) -> (76.2, 51.6382)
  line L1918 (76.158, 52.243) -> (76.158, 51.643)
  line L1919 (22.8092, 28.702) -> (22.8092, 29.718)
  line L1920 (23.414, 29.76) -> (22.814, 29.76)
  line L1921 (77.043, 47.54) -> (77.043, 46.44)
  line L1922 (20.151, 33.736) -> (21.251, 33.736)
  line L1923 (21.209, 33.7312) -> (20.193, 33.7312)
  line L1924 (32.308, 51.534) -> (33.408, 51.534)
  line L1925 (22.814, 29.76) -> (22.814, 28.66)
  line L1926 (33.366, 51.5292) -> (32.35, 51.5292)
  line L1927 (23.4188, 28.702) -> (22.8092, 28.702)
  line L1928 (22.8092, 29.718) -> (23.4188, 29.718)
  line L1929 (20.193, 33.7312) -> (20.193, 34.3408)
  line L1930 (22.8092, 28.702) -> (22.8092, 29.718)
  line L1931 (23.4188, 29.085) -> (23.4188, 29.335)
  line L1932 (22.1488, 29.085) -> (22.1488, 29.335)
  line L1933 (77.6478, 47.498) -> (77.6478, 46.482)
  line L1934 (21.5392, 29.718) -> (22.1488, 29.718)
  line L1935 (21.251, 34.336) -> (20.151, 34.336)
  line L1936 (22.1488, 29.335) -> (21.5392, 29.335)
  line L1937 (22.8092, 29.085) -> (23.4188, 29.085)
  line L1938 (23.414, 28.66) -> (23.414, 29.76)
  line L1939 (20.151, 34.336) -> (20.151, 33.736)
  line L1940 (23.4188, 29.718) -> (23.4188, 28.702)
  line L1941 (76.583, 51.6382) -> (76.833, 51.6382)
  line L1942 (22.814, 28.66) -> (23.414, 28.66)
  line L1943 (22.8092, 29.335) -> (22.8092, 29.085)
  line L1944 (32.35, 52.1388) -> (33.366, 52.1388)
  line L1945 (76.833, 51.6382) -> (76.833, 52.2478)
  line L1946 (33.408, 53.404) -> (32.308, 53.404)
  line L1947 (22.8092, 29.718) -> (23.4188, 29.718)
  line L1948 (21.209, 33.7312) -> (20.193, 33.7312)
  line L1949 (22.1488, 28.702) -> (21.5392, 28.702)
  line L1950 (33.366, 52.7992) -> (32.35, 52.7992)
  line L1951 (21.209, 34.3408) -> (21.209, 33.7312)
  line L1952 (21.5392, 28.702) -> (21.5392, 29.718)
  line L1953 (22.1488, 29.718) -> (22.1488, 28.702)
  line L1954 (83.843, 27.145) -> (83.543, 27.145)
  line L1955 (21.5392, 29.335) -> (21.5392, 29.085)
  line L1956 (77.0382, 46.482) -> (77.0382, 47.498)
  line L1957 (77.216, 52.2478) -> (77.216, 51.6382)
  line L1958 (76.833, 52.2478) -> (76.583, 52.2478)
  line L1959 (23.4188, 29.718) -> (23.4188, 28.702)
  line L1960 (20.576, 34.3408) -> (20.576, 33.7312)
  line L1961 (23.4188, 28.702) -> (22.8092, 28.702)
  line L1962 (21.544, 28.66) -> (22.144, 28.66)
  line L1963 (21.544, 29.76) -> (21.544, 28.66)
  line L1964 (21.5392, 29.085) -> (22.1488, 29.085)
  line L1965 (21.251, 33.736) -> (21.251, 34.336)
  line L1966 (76.2, 52.2478) -> (77.216, 52.2478)
  line L1967 (21.5392, 29.718) -> (22.1488, 29.718)
  line L1968 (83.5152, 26.3398) -> (83.8708, 26.3398)
  line L1969 (22.144, 29.76) -> (21.544, 29.76)
  line L1970 (77.216, 52.2478) -> (77.216, 51.6382)
  line L1971 (22.1488, 28.702) -> (21.5392, 28.702)
  line L1972 (76.2, 51.6382) -> (76.2, 52.2478)
  line L1973 (22.1488, 29.718) -> (22.1488, 28.702)
  line L1974 (22.144, 28.66) -> (22.144, 29.76)
  line L1975 (23.4188, 29.335) -> (22.8092, 29.335)
  line L1976 (77.258, 52.243) -> (76.158, 52.243)
  line L1977 (77.216, 51.6382) -> (76.2, 51.6382)
  line L1978 (76.2, 51.6382) -> (76.2, 52.2478)
  line L1979 (76.2, 52.2478) -> (77.216, 52.2478)
  line L1980 (21.5392, 28.702) -> (21.5392, 29.718)
  line L1981 (32.733, 53.4088) -> (32.733, 52.7992)
  line L1982 (20.826, 34.3408) -> (20.576, 34.3408)
  line L1983 (32.983, 51.5292) -> (32.983, 52.1388)
  line L1984 (35.435, 34.8862) -> (35.435, 35.4958)
  line L1985 (33.366, 52.7992) -> (32.35, 52.7992)
  line L1986 (20.576, 33.7312) -> (20.826, 33.7312)
  line L1987 (33.366, 51.5292) -> (32.35, 51.5292)
  line L1988 (56.818, 14.4648) -> (56.818, 13.8552)
  line L1989 (57.9882, 55.626) -> (58.5978, 55.626)
  line L1990 (27.2542, 51.181) -> (27.8638, 51.181)
  line L1991 (33.366, 52.1388) -> (33.366, 51.5292)
  line L1992 (32.983, 53.4088) -> (32.733, 53.4088)
  line L1993 (56.818, 13.8552) -> (55.802, 13.8552)
  line L1994 (32.983, 52.7992) -> (32.983, 53.4088)
  line L1995 (55.802, 13.8552) -> (55.802, 14.4648)
  line L1996 (58.5978, 54.61) -> (57.9882, 54.61)
  line L1997 (32.35, 52.1388) -> (33.366, 52.1388)
  line L1998 (32.35, 53.4088) -> (33.366, 53.4088)
  line L1999 (32.35, 53.4088) -> (33.366, 53.4088)
  line L2000 (27.859, 51.223) -> (27.259, 51.223)
  line L2001 (57.993, 54.568) -> (58.593, 54.568)
  line L2002 (20.193, 33.7312) -> (20.193, 34.3408)
  line L2003 (56.86, 13.86) -> (56.86, 14.46)
  line L2004 (56.185, 13.8552) -> (56.435, 13.8552)
  line L2005 (35.818, 35.4958) -> (35.818, 34.8862)
  line L2006 (58.5978, 55.626) -> (58.5978, 54.61)
  line L2007 (33.408, 52.804) -> (33.408, 53.404)
  line L2008 (35.818, 34.8862) -> (34.802, 34.8862)
  line L2009 (27.2542, 51.181) -> (27.8638, 51.181)
  line L2010 (32.35, 51.5292) -> (32.35, 52.1388)
  line L2011 (32.733, 51.5292) -> (32.983, 51.5292)
  line L2012 (32.733, 52.1388) -> (32.733, 51.5292)